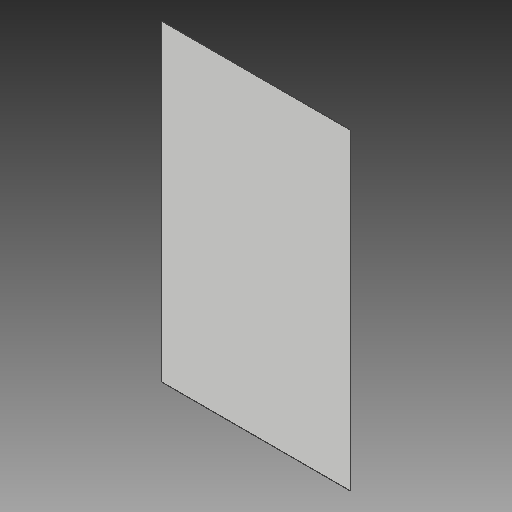
# Autodesk Inventor part: chapa_referencia_tampa_gabinete
Saved by Autodesk Inventor 2018 (Build 220112000, 112)
## iProperties
Created: 2018-05-16
Part Number: chapa_referencia_tampa_gabinete
Material: Genérico
Document SubType Name: Chapa de metal
Designer: Usuario
Density: 1 g/cm^3
Sheet Metal Rule: Padrão_mm
Appearance: Padrão
Author: Usuario
Autodesk Inventor part; units mm, degrees
ref_plane "YZ Plane" through (0, 0, 0) normal (1, 0, 0) x (0, 1, 0)
ref_plane "XZ Plane" through (0, 0, 0) normal (0, 1, 0) x (-1, 0, 0)
ref_plane "XY Plane" through (0, 0, 0) normal (0, 0, 1) x (1, 0, 0)
sketch "Esboço1" plane through (0, 0, 0) normal (0, 0, 1) x (1, 0, 0)
  line L0 (-117.1185, 282.2911) -> (152.8815, 282.2911) construction
  line L1 (0, 0) -> (0, -220) construction
  line L2 (0, -220) -> (160, -220) construction
  line L3 (160, -220) -> (160, 330.078) construction
  line L4 (160, 330.078) -> (-170, 330.078) construction
  line L5 (-170, 330.078) -> (-170, -220) construction
  line L6 (-170, -220) -> (0, -220) construction
  line L7 (160, 330.078) -> (-170, -220) construction
  line L8 (160, -220) -> (-170, 330.078) construction
  line L9 (-172, 332.039) -> (162, 332.039)
  line L10 (162, 332.039) -> (162, -221.961)
  line L11 (162, -221.961) -> (-172, -221.961)
  line L12 (-172, -221.961) -> (-172, 332.039)
  line L13 (-172, 332.039) -> (162, -221.961) construction
  line L14 (162, 332.039) -> (-172, -221.961) construction
  point P0 (-5, 55.039)
  dimension "d0" = 220
  dimension "d1" = 160
  dimension "d2" = 330
  dimension "d3" = 334
  dimension "d4" = 554
  measures "d0" distance of L1.start L1.end
  measures "d1" distance of L1.end L2.end
  measures "d2" distance of L3.end L4.end
  measures "d3" distance of L10.end L11.end
  measures "d4" distance of L9.end L10.end
extrude "Placa1" add sketch "Esboço1" along normal blind 0.5
equation "\"Raio_vergadura\" = Espessura"
equation "\"Largura_alívio_de_vergadura\" = Espessura"
equation "\"Profundidade_alívio_de_vergadura\" = 0.5 * Espessura"
equation "\"Tamanho_alívio_de_dobra\" = 4 * Espessura"
equation "\"Remanescente_mínimo\" = 2 * Espessura"
equation "\"Raiodetransição\" = Raio_vergadura"
equation "\"Tamanho_de_raio_de_Jacobi\" = Raio_vergadura"
equation "\"TamanhoFolga\" = Espessura"
